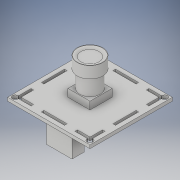
# Autodesk Inventor part: camera
Saved by Autodesk Inventor 2018 (Build 220112000, 112)
## iProperties
Created: 2020-03-27
Part Number: camera
Material: Generic
Document SubType Name: Modeling
Designer: natha
Density: 1 g/cm^3
Appearance: Default
Author: natha
Autodesk Inventor part; units mm, degrees
ref_plane "YZ Plane" through (0, 0, 0) normal (1, 0, 0) x (0, 1, 0)
ref_plane "XZ Plane" through (0, 0, 0) normal (0, 1, 0) x (-1, 0, 0)
ref_plane "XY Plane" through (0, 0, 0) normal (0, 0, 1) x (1, 0, 0)
sketch "Sketch1" plane through (0, 0, 0) normal (0, 1, 0) x (-1, 0, 0)
  line L0 (0, 0) -> (32.1, 0)
  line L1 (32.1, 0) -> (32.1, -32.1)
  line L2 (32.1, -32.1) -> (0, -32.1)
  line L3 (0, -32.1) -> (0, 0)
  circle A0 centre (30.6, -30.6) radius 1.125
  circle A1 centre (1.5, -30.6) radius 1.125
  circle A2 centre (1.5, -1.5) radius 1.125
  circle A3 centre (30.6, -1.5) radius 1.125
  line L4 (30.6, -2.625) -> (24.6, -2.625)
  line L5 (24.6, -2.625) -> (24.6, -1.625)
  line L6 (24.6, -1.625) -> (30.6, -1.625)
  line L7 (30.6, -1.625) -> (30.6, -2.625)
  line L8 (29.475, -1.5) -> (30.475, -1.5)
  line L9 (30.475, -1.5) -> (30.475, -7.5)
  line L10 (30.475, -7.5) -> (29.475, -7.5)
  line L11 (29.475, -7.5) -> (29.475, -1.5)
  line L12 (1.5, -2.625) -> (7.5, -2.625)
  line L13 (7.5, -2.625) -> (7.5, -1.625)
  line L14 (7.5, -1.625) -> (1.5, -1.625)
  line L15 (1.5, -1.625) -> (1.5, -2.625)
  line L16 (2.625, -1.5) -> (1.625, -1.5)
  line L17 (1.625, -1.5) -> (1.625, -7.5)
  line L18 (1.625, -7.5) -> (2.625, -7.5)
  line L19 (2.625, -7.5) -> (2.625, -1.5)
  line L20 (1.5, -29.475) -> (7.5, -29.475)
  line L21 (7.5, -29.475) -> (7.5, -30.475)
  line L22 (7.5, -30.475) -> (1.5, -30.475)
  line L23 (1.5, -30.475) -> (1.5, -29.475)
  line L24 (2.625, -30.6) -> (1.625, -30.6)
  line L25 (1.625, -30.6) -> (1.625, -24.6)
  line L26 (1.625, -24.6) -> (2.625, -24.6)
  line L27 (2.625, -24.6) -> (2.625, -30.6)
  line L28 (30.6, -29.475) -> (24.6, -29.475)
  line L29 (24.6, -29.475) -> (24.6, -30.475)
  line L30 (24.6, -30.475) -> (30.6, -30.475)
  line L31 (30.6, -30.475) -> (30.6, -29.475)
  line L32 (29.475, -30.6) -> (30.475, -30.6)
  line L33 (30.475, -30.6) -> (30.475, -24.6)
  line L34 (30.475, -24.6) -> (29.475, -24.6)
  line L35 (29.475, -24.6) -> (29.475, -30.6)
  line L36 (20.55, -1.625) -> (11.55, -1.625)
  line L37 (11.55, -1.625) -> (11.55, -2.625)
  line L38 (11.55, -2.625) -> (20.55, -2.625)
  line L39 (20.55, -2.625) -> (20.55, -1.625)
  line L40 (20.55, -29.475) -> (11.55, -29.475)
  line L41 (11.55, -29.475) -> (11.55, -30.475)
  line L42 (11.55, -30.475) -> (20.55, -30.475)
  line L43 (20.55, -30.475) -> (20.55, -29.475)
  line L44 (30.475, -11.55) -> (29.475, -11.55)
  line L45 (29.475, -11.55) -> (29.475, -20.55)
  line L46 (29.475, -20.55) -> (30.475, -20.55)
  line L47 (30.475, -20.55) -> (30.475, -11.55)
  line L48 (2.625, -11.55) -> (1.625, -11.55)
  line L49 (1.625, -11.55) -> (1.625, -20.55)
  line L50 (1.625, -20.55) -> (2.625, -20.55)
  line L51 (2.625, -20.55) -> (2.625, -11.55)
  dimension "d0" = 32.1
  dimension "d1" = 32.1
  dimension "d2" = 2.25
  dimension "d3" = 2.25
  dimension "d4" = 2.25
  dimension "d5" = 2.25
  dimension "d6" = 1.5
  dimension "d7" = 1.5
  dimension "d8" = 1.5
  dimension "d9" = 1.5
  dimension "d10" = 1.5
  dimension "d11" = 1.5
  dimension "d12" = 1.5
  dimension "d13" = 1.5
  dimension "d14" = 6
  dimension "d15" = 1
  dimension "d16" = 1
  dimension "d17" = 6
  dimension "d18" = 6
  dimension "d19" = 1
  dimension "d20" = 1
  dimension "d21" = 6
  dimension "d22" = 6
  dimension "d23" = 1
  dimension "d24" = 1
  dimension "d25" = 6
  dimension "d26" = 6
  dimension "d27" = 1
  dimension "d28" = 1
  dimension "d29" = 6
  dimension "d30" = 9
  dimension "d31" = 1
  dimension "d32" = 4.05
  dimension "d33" = 1
  dimension "d34" = 9
  dimension "d35" = 1
  dimension "d36" = 9
  dimension "d37" = 4.05
  dimension "d38" = 4.05
  constraints: 104 end point, 26 parallel, 13 horizontal, 13 perpendicular, 8 point on circle, 4 centre point, 3 point on line
  measures "d0" distance of L1.end L2.end
  measures "d1" distance of L0.end L1.end
  measures "d2" diameter of A0
  measures "d3" diameter of A1
  measures "d4" diameter of A2
  measures "d5" diameter of A3
  measures "d6" distance from line of L1 A3.centre
  measures "d7" distance from line of L0 A3.centre
  measures "d8" distance from line of L1 A0.centre
  measures "d9" distance from line of L2 A0.centre
  measures "d10" distance from line of L2 A1.centre
  measures "d11" distance from line of L3 A1.centre
  measures "d12" distance from line of L3 A2.centre
  measures "d13" distance from line of L0 A2.centre
  measures "d14" distance of L5.end L6.end
  measures "d15" distance of L4.end L5.end
  measures "d16" distance of L9.end L10.end
  measures "d17" distance of L8.end L9.end
  measures "d18" distance of L14.end L13.end
  measures "d19" distance of L13.end L12.end
  measures "d20" distance of L18.end L17.end
  measures "d21" distance of L17.end L16.end
  measures "d22" distance of L21.end L22.end
  measures "d23" distance of L20.end L21.end
  measures "d24" distance of L25.end L26.end
  measures "d25" distance of L24.end L25.end
  measures "d26" distance of L30.end L29.end
  measures "d27" distance of L29.end L28.end
  measures "d28" distance of L34.end L33.end
  measures "d29" distance of L33.end L32.end
  measures "d30" distance of L38.end L37.end
  measures "d31" distance of L37.end L36.end
  measures "d32" distance between parallel lines of L5 L39
  measures "d33" distance of L41.end L40.end
  measures "d34" distance of L45.end L44.end
  measures "d35" distance of L50.end L49.end
  measures "d36" distance of L49.end L48.end
  measures "d37" distance between parallel lines of L48 L18
  measures "d38" distance between parallel lines of L44 L10
extrude "Extrusion1" add sketch "Sketch1" along normal blind 1.3
sketch "Sketch2" plane through (0, 1.3, 0) normal (0, 1, 0) x (1, 0, 0)
  line L0 (-20.35, 11.75) -> (-11.75, 11.75)
  line L1 (-11.75, 11.75) -> (-11.75, 20.35)
  line L2 (-11.75, 20.35) -> (-20.35, 20.35)
  line L3 (-20.35, 20.35) -> (-20.35, 11.75)
  line L4 (-32.1, 0) -> (0, 0) projected
  line L5 (-32.1, 32.1) -> (-32.1, 0) projected
  dimension "d41" = 8.6
  dimension "d42" = 8.6
  dimension "d43" = 11.75
  dimension "d44" = 11.75
  constraints: 8 end point, 2 parallel, 1 horizontal, 1 perpendicular
  measures "d41" distance of L2.end L1.end
  measures "d42" distance of L1.end L0.end
  measures "d43" distance between parallel lines of L4 L0
  measures "d44" distance between parallel lines of L5 L3
extrude "Extrusion2" add sketch "Sketch2" along normal blind 3
sketch "Sketch3" plane through (0, 4.3, 0) normal (0, 1, 0) x (1, 0, 0)
  circle A0 centre (-16.05, 16.05) radius 4
  line L0 (-20.35, 20.35) -> (-20.35, 11.75) projected
  line L1 (-11.75, 20.35) -> (-20.35, 20.35) projected
  point P0 (0, 0)
  dimension "d47" = 8
  dimension "d48" = 4.3
  dimension "d49" = 4.3
  constraints: 1 centre point
  measures "d47" diameter of A0
  measures "d48" distance from line of L0 A0.centre
  measures "d49" distance from line of L1 A0.centre
extrude "Extrusion3" add sketch "Sketch3" along normal blind 6.7
sketch "Sketch4" plane through (-16.05, 11, -16.05) normal (0, 1, 0) x (1, 0, 0)
  circle A0 centre (0, 0) radius 5
  point P0 (16.05, -16.05)
  dimension "d52" = 10
  constraints: 1 centre point
  measures "d52" diameter of A0
extrude "Extrusion4" add sketch "Sketch4" along normal blind 4.5
sketch "Sketch5" plane through (0, 0, 0) normal (0, -1, 0) x (1, 0, 0)
  line L0 (-18, -1) -> (-8, -1)
  line L1 (-8, -1) -> (-8, -5.7)
  line L2 (-8, -5.7) -> (-18, -5.7)
  line L3 (-18, -5.7) -> (-18, -1)
  line L4 (0, -32.1) -> (0, 0) projected
  line L5 (0, 0) -> (-32.1, 0) projected
  dimension "d55" = 10
  dimension "d56" = 4.7
  dimension "d57" = 8
  dimension "d58" = 1
  constraints: 8 end point, 2 parallel, 1 horizontal, 1 perpendicular
  measures "d55" distance of L1.end L2.end
  measures "d56" distance of L0.end L1.end
  measures "d57" distance between parallel lines of L4 L1
  measures "d58" distance between parallel lines of L5 L0
extrude "Extrusion5" add sketch "Sketch5" along normal blind 8
sketch "Sketch6" plane through (-16.05, 15.5, -16.05) normal (0, 1, 0) x (1, 0, 0)
  circle A0 centre (0, 0) radius 3.5
  point P0 (16.05, -16.05)
  dimension "d61" = 7
  constraints: 1 centre point
  measures "d61" diameter of A0
extrude "Extrusion6" cut sketch "Sketch6" against normal blind 0.5
fillet "Fillet1" radius 2 1 edges at (-19.55, 15.5, -16.05)
body "Solid1"
